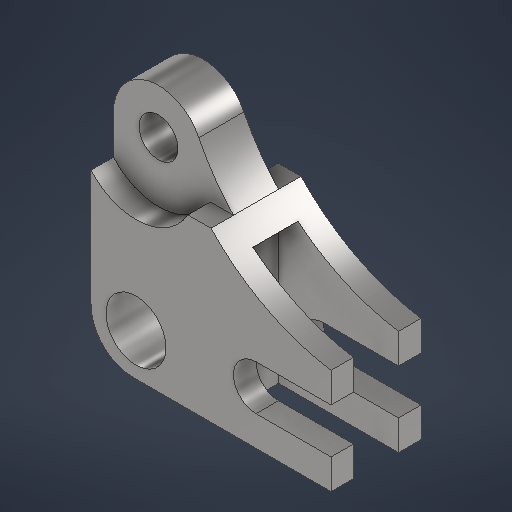
# Autodesk Inventor part: ensayo 8
Saved by Autodesk Inventor 2026.2 (Build 302298000, 298)
## iProperties
Created: 2025-12-22
Part Number: ensayo 8
Material: Acero inoxidable
Document SubType Name: Modeling
Designer: vicho
Mass: 644.593 g
Surface Area: 204.351 cm^2
Volume: 80.5741 cm^3
Density: 8 g/cm^3
Appearance: Semipulido
Author: vicho
Autodesk Inventor part; units mm, degrees
ref_plane "YZ Plane" through (0, 0, 0) normal (1, 0, 0) x (0, 1, 0)
ref_plane "XZ Plane" through (0, 0, 0) normal (0, 1, 0) x (-1, 0, 0)
ref_plane "XY Plane" through (0, 0, 0) normal (0, 0, 1) x (1, 0, 0)
sketch "Boceto1" plane through (0, 0, 0) normal (0, 0, 1) x (1, 0, 0)
  line L0 (0, 50) -> (0, -50) construction
  line L1 (-50, 0) -> (50, 0) construction
  line L2 (-50, -52) -> (50, -52) construction
  circle A0 centre (0, -52) radius 10
  circle A1 centre (0, 0) radius 6.5
  arc A2 (13.4711, 6.5977) -> (-15, 0) centre (0, 0) ccw
  arc A3 (-15, -13.2288) -> (17.3205, -10) centre (0, 0) ccw
  line L3 (17.3205, -10) -> (25, -10)
  line L4 (40, -56) -> (65, -56)
  line L5 (65, -56) -> (65, -66)
  line L6 (65, -66) -> (40, -66)
  line L7 (-15, 0) -> (-15, -66)
  line L8 (65, 25.2383) -> (65, -76.5705) construction
  line L9 (40, -66) -> (-15, -66)
  line L10 (40, -41) -> (65, -41)
  arc A4 (40, -41) -> (40, -56) centre (40, -48.5) ccw
  line L11 (65, -41) -> (65, -31)
  line L12 (25, 28.6395) -> (25, -70.532) construction
  arc A5 (25, -10) -> (65, -31) centre (75.7977, 38.1622) ccw
  arc A6 (13.4711, 6.5977) -> (25, -10) centre (73.5302, 36.0124) ccw
  point P0 (0, 0)
  point P1 (17.3859, -10)
  point P2 (65, -61)
  point P3 (40, -61)
  point P4 (52.5, -41)
  dimension "d0" = 100
  dimension "d1" = 100
  dimension "d2" = 52
  dimension "d3" = 100
  dimension "d4" = 20
  dimension "d5" = 13
  dimension "d6" = 15
  dimension "d7" = 20
  dimension "d8" = 10
  dimension "d9" = 56
  dimension "d10" = 10
  dimension "d11" = 25
  dimension "d12" = 80
  dimension "d14" = 15
  dimension "d15" = 7.5
  dimension "d16" = 7.5
  dimension "d17" = 25
  dimension "d18" = 10
  dimension "d19" = 40
  dimension "d20" = 25
  dimension "d21" = 80
  dimension "d22" = 70
  dimension "d23" = 7.6141
  constraints: 26 end point, 10 point on circle, 7 centre point, 7 midpoint, 7 point on line, 5 coincident, 5 horizontal, 4 vertical, 3 symmetric about line, 2 perpendicular, 2 tangent, 1 parallel
  measures "d0" distance of L0.end L0.start
  measures "d1" distance of L1.end L1.start
  measures "d2" distance of point (0, 0) point (0, -52)
  measures "d3" distance of L2.end L2.start
  measures "d4" diameter of A0
  measures "d5" diameter of A1
  measures "d6" radius of A2
  measures "d7" radius of A3
  measures "d8" distance from line of L3 point (0, 0)
  measures "d9" distance from line of L6 point (17.386, -10)
  measures "d10" distance between parallel lines of L6 L4
  measures "d11" distance of point (65, -61) point (40, -61)
  measures "d12" distance between parallel lines of L8 L7
  measures "d14" distance from line of L4 point (52.5, -41)
  measures "d15" distance from line of L10 point (40, -48.5)
  measures "d16" radius of A4
  measures "d17" distance of L10.end L10.start
  measures "d18" distance of L10.end L11.end
  measures "d19" distance between parallel lines of L12 L7
  measures "d20" distance from line of L4.start L8
  measures "d21" distance between parallel lines of L5 L7
  measures "d22" radius of A5
  measures "d23" distance of L3.end point (17.386, -10)
extrude "Extrusión1" add sketch "Boceto1" along normal mid plane 15 contours A6 L3 A3 L7 A2
extrude "Extrusión2" add sketch "Boceto1" along normal mid plane 30 contours A5 L11 L10 A4 L4 L5 L6 L9 L7 A3 L3
fillet "Empalme1" radius 14 1 edges at (-15, -66, 0)
sketch "Boceto2" plane through (65, -66, -15) normal (0, -1, 0) x (1, 0, 0)
  line L0 (0, 0) -> (0, 30) projected
  line L1 (0, 22.5) -> (-40, 22.5)
  line L2 (-40, 22.5) -> (-40, 7.5)
  line L3 (-40, 7.5) -> (0, 7.5)
  line L4 (0, 7.5) -> (0, 22.5)
  line L5 (38.7229, 15) -> (-93.8867, 15) construction
  point P0 (-65, 15)
  point P1 (0, 7.5)
  dimension "d29" = 40
  dimension "d30" = 15
  dimension "d31" = 15
  dimension "d32" = 132.6097
  dimension "d33" = 38.7229
  constraints: 10 end point, 3 parallel, 1 horizontal, 1 perpendicular, 1 point on line, 1 symmetric about line
  measures "d29" distance of L1.end L1.start
  measures "d30" distance of L1.end L2.end
  measures "d31" distance from line of L0.end L5
  measures "d32" distance of L5.end L5.start
  measures "d33" distance from line of L5.start L0
extrude "Extrusión3" cut sketch "Boceto2" against normal blind 50
